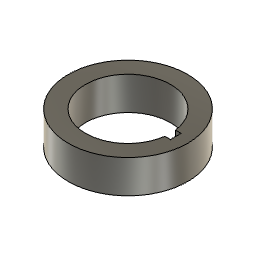
Slit Adjust Pully v1 (Autodesk Fusion 360 design; units mm, degrees)
Autodesk Fusion 360 part; units mm, degrees
sketch "Sketch1" plane through (0, 0, 0) normal (0, 0, 1) x (1, 0, 0)
  circle A0 centre (0, 0) radius 16
  line L0 (0, 0) -> (16, 0)
  line L1 (15.8745, -2) -> (18, -2)
  line L2 (18, -2) -> (18, 2)
  line L3 (18, 2) -> (15.8745, 2)
  circle A1 centre (0, 0) radius 22.5
  dimension "d1" = 32
  constraint coincident A0.centre L0.start
  constraint coincident A0 L0.end
  constraint horizontal L0
  constraint coincident A0 L1.start
  constraint perpendicular L1 L2
  constraint coincident A0 L3.end
  constraint concentric A0 A1
  measures "d1" diameter of A0
extrude "Extrude1" add sketch "Sketch1" along normal blind 12.5
